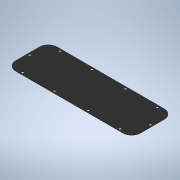
# Autodesk Inventor part: CAD_FPL_1050.000
Saved by Autodesk Inventor 2021 (Build 250183000, 183)
## iProperties
Created: 2025-07-29
Part Number: CAD_FPL_1050.000
Material: Generic
Catalog Web Link: www.cadenas.de
Description: Gland plate AX-Compact enclosures
Vendor: RITTAL
Document SubType Name: Modeling
Designer: psAdmin
Manufacturer: RITTAL
Mass: 97.9753 g
Surface Area: 1326.79 cm^2
Volume: 97.9753 cm^3
Density: 1 g/cm^3
Appearance: PSOLRGB-175-175-175
Category: PARTsolutions
Company: RITTAL
Title: CAD_FPL_1050.000
Author: Cadenas PARTsolutions
Comments: Compact enclosures
PSOL_IDENT_0: {$CADENAS_DATA/23d-libs/rittal/schaltschranksys/ausbauteile_cad/flanschplatten/ae_2_0_sep_fpl.prj},1
PSOL_IDENT_1: 81 {VTYP=3D},{NB=CAD_FPL_1050.000},{LINA=CAD_FPL_1050.000},{NN=Gland plate AX},{DATE=28.04.2025 21:1
PSOL_IDENT_2: 0:23},{GEOMDATE=11.04.2025 07:45:17},{VERSION=},{LINEID=180},{WBVAR=},{WBNUMERIC=}  {NB=CAD_FPL_1050
PSOL_IDENT_3: .000},{LINA=CAD_FPL_1050.000},{KT=DUMMY},{BEST=CAD_FPL_1050.000},{DETAIL=1},{VERS=4},{D=447},{E=149}
PSOL_IDENT_4: ,{BEZ1=Neues Kompaktgehäuse},{BEZ2=Stahlblech},{BEZ3=eintürig},{TUER=1},{B=500},{H=500},{T=210},{F=4
PSOL_IDENT_5: 50},{G=475},{B1=500},{B3=460.000},{B4=383.000},{B5=411.000},{BB5=0.000},{H1=500},{H3=460.000},{H4=85
PSOL_IDENT_6: .000},{H5=113.000},{HH5=4.000},{T5=93.500},{R1=31.000},{R2=8.000},{T1=210},{F1=450},{G1=475},{ST=MIN
PSOL_IDENT_7: },{VERS3=0},{CNSECLASS51=27-18-01-02},{CNSECLASS70=27-18-01-01},{CNSECLASS80=27-18-01-01},{CNSETIM40=
PSOL_IDENT_8: EC000261},{S=1.25},{W=500.000},{W1=456.500},{W2=400.000},{HH=500.000},{HH1=456.500},{HH2=450.000},{H
PSOL_IDENT_9: H3=375.000},{D1=204.300},{VERS1=1}
NB: CAD_FPL_1050.000
NN: Gland plate AX
NT: Compact enclosures
NBSYN: $BEST.
LINA: CAD_FPL_1050.000
CATALOG: Rittal
BEST: CAD_FPL_1050.000
D: 447
E: 149
SUPPLIER: RITTAL
ARTICLENO: CAD_FPL_1050.000
BOMINFO: CAD_FPL_1050.000
CREATOR: CADENAS GmbH
Autodesk Inventor part; units mm, degrees
(part 1 of 3)
sketch "Sketch_4" plane through (0, 0, 0) normal (0, 1, 0) x (1, 0, 0)
  arc A0 (-223.5, -42.5) -> (-191.5, -74.5) centre (-191.5, -42.5) ccw
  line L0 (-191.5, -74.5) -> (191.5, -74.5)
  arc A1 (191.5, -74.5) -> (223.5, -42.5) centre (191.5, -42.5) ccw
  line L1 (223.5, -42.5) -> (223.5, 42.5)
  arc A2 (223.5, 42.5) -> (191.5, 74.5) centre (191.5, 42.5) ccw
  line L2 (191.5, 74.5) -> (-191.5, 74.5)
  arc A3 (-191.5, 74.5) -> (-223.5, 42.5) centre (-191.5, 42.5) ccw
  line L3 (-223.5, 42.5) -> (-223.5, -42.5)
  circle A4 centre (215.5, 0) radius 3.6
  circle A5 centre (174, -66.5) radius 3.6
  circle A6 centre (174, 66.5) radius 3.6
  circle A7 centre (60, -66.5) radius 3.6
  circle A8 centre (60, 66.5) radius 3.6
  circle A9 centre (-60, -66.5) radius 3.6
  circle A10 centre (-60, 66.5) radius 3.6
  circle A11 centre (-174, -66.5) radius 3.6
  circle A12 centre (-174, 66.5) radius 3.6
  circle A13 centre (-215.5, 0) radius 3.6
  constraints: 14 centre point, 8 end point, 8 point on circle
extrude "Extrusion1" add sketch "Sketch_4" along normal blind 1.5
ref_plane "FP_XY" through (0, 0, 0) normal (0, -1, 0) x (1, 0, 0)
ref_plane "FP_YZ" through (0, 0, 0) normal (1, 0, 0) x (0, 0, 1)
ref_plane "FP_ZX" through (0, 0, 0) normal (0, 0, 1) x (0, -1, 0)
ref_plane "to_Bolt_1_XY" through (-250, 0, -250) normal (0, 1, 0) x (1, 0, 0)
ref_plane "to_Bolt_1_YZ" through (-250, 0, -250) normal (1, 0, 0) x (0, 0, -1)
ref_plane "to_Bolt_1_ZX" through (-250, 0, -250) normal (0, 0, -1) x (0, 1, 0)
ref_plane "to_Bolt_1_1_XY" through (-244, 0, -250) normal (0, 1, 0) x (1, 0, 0)
ref_plane "to_Bolt_1_1_YZ" through (-244, 0, -250) normal (1, 0, 0) x (0, 0, -1)
ref_plane "to_Bolt_1_1_ZX" through (-244, 0, -250) normal (0, 0, -1) x (0, 1, 0)
ref_plane "to_Bolt_1_10_XY" through (-228.4689, 0, -250) normal (0, 1, 0) x (1, 0, 0)
ref_plane "to_Bolt_1_10_YZ" through (-228.4689, 0, -250) normal (1, 0, 0) x (0, 0, -1)
ref_plane "to_Bolt_1_10_ZX" through (-228.4689, 0, -250) normal (0, 0, -1) x (0, 1, 0)
ref_plane "to_Bolt_1_100_XY" through (-13.1579, 0, -250) normal (0, 1, 0) x (1, 0, 0)
ref_plane "to_Bolt_1_100_YZ" through (-13.1579, 0, -250) normal (1, 0, 0) x (0, 0, -1)
ref_plane "to_Bolt_1_100_ZX" through (-13.1579, 0, -250) normal (0, 0, -1) x (0, 1, 0)
ref_plane "to_Bolt_1_101_XY" through (-10.7656, 0, -250) normal (0, 1, 0) x (1, 0, 0)
ref_plane "to_Bolt_1_101_YZ" through (-10.7656, 0, -250) normal (1, 0, 0) x (0, 0, -1)
ref_plane "to_Bolt_1_101_ZX" through (-10.7656, 0, -250) normal (0, 0, -1) x (0, 1, 0)
ref_plane "to_Bolt_1_102_XY" through (-8.3732, 0, -250) normal (0, 1, 0) x (1, 0, 0)
ref_plane "to_Bolt_1_102_YZ" through (-8.3732, 0, -250) normal (1, 0, 0) x (0, 0, -1)
ref_plane "to_Bolt_1_102_ZX" through (-8.3732, 0, -250) normal (0, 0, -1) x (0, 1, 0)
ref_plane "to_Bolt_1_103_XY" through (-5.9809, 0, -250) normal (0, 1, 0) x (1, 0, 0)
ref_plane "to_Bolt_1_103_YZ" through (-5.9809, 0, -250) normal (1, 0, 0) x (0, 0, -1)
ref_plane "to_Bolt_1_103_ZX" through (-5.9809, 0, -250) normal (0, 0, -1) x (0, 1, 0)
ref_plane "to_Bolt_1_104_XY" through (-3.5885, 0, -250) normal (0, 1, 0) x (1, 0, 0)
ref_plane "to_Bolt_1_104_YZ" through (-3.5885, 0, -250) normal (1, 0, 0) x (0, 0, -1)
ref_plane "to_Bolt_1_104_ZX" through (-3.5885, 0, -250) normal (0, 0, -1) x (0, 1, 0)
ref_plane "to_Bolt_1_105_XY" through (-1.1962, 0, -250) normal (0, 1, 0) x (1, 0, 0)
ref_plane "to_Bolt_1_105_YZ" through (-1.1962, 0, -250) normal (1, 0, 0) x (0, 0, -1)
ref_plane "to_Bolt_1_105_ZX" through (-1.1962, 0, -250) normal (0, 0, -1) x (0, 1, 0)
ref_plane "to_Bolt_1_106_XY" through (1.1962, 0, -250) normal (0, 1, 0) x (1, 0, 0)
ref_plane "to_Bolt_1_106_YZ" through (1.1962, 0, -250) normal (1, 0, 0) x (0, 0, -1)
ref_plane "to_Bolt_1_106_ZX" through (1.1962, 0, -250) normal (0, 0, -1) x (0, 1, 0)
ref_plane "to_Bolt_1_107_XY" through (3.5885, 0, -250) normal (0, 1, 0) x (1, 0, 0)
ref_plane "to_Bolt_1_107_YZ" through (3.5885, 0, -250) normal (1, 0, 0) x (0, 0, -1)
ref_plane "to_Bolt_1_107_ZX" through (3.5885, 0, -250) normal (0, 0, -1) x (0, 1, 0)
ref_plane "to_Bolt_1_108_XY" through (5.9809, 0, -250) normal (0, 1, 0) x (1, 0, 0)
ref_plane "to_Bolt_1_108_YZ" through (5.9809, 0, -250) normal (1, 0, 0) x (0, 0, -1)
ref_plane "to_Bolt_1_108_ZX" through (5.9809, 0, -250) normal (0, 0, -1) x (0, 1, 0)
ref_plane "to_Bolt_1_109_XY" through (8.3732, 0, -250) normal (0, 1, 0) x (1, 0, 0)
ref_plane "to_Bolt_1_109_YZ" through (8.3732, 0, -250) normal (1, 0, 0) x (0, 0, -1)
ref_plane "to_Bolt_1_109_ZX" through (8.3732, 0, -250) normal (0, 0, -1) x (0, 1, 0)
ref_plane "to_Bolt_1_11_XY" through (-226.0766, 0, -250) normal (0, 1, 0) x (1, 0, 0)
ref_plane "to_Bolt_1_11_YZ" through (-226.0766, 0, -250) normal (1, 0, 0) x (0, 0, -1)
ref_plane "to_Bolt_1_11_ZX" through (-226.0766, 0, -250) normal (0, 0, -1) x (0, 1, 0)
ref_plane "to_Bolt_1_110_XY" through (10.7656, 0, -250) normal (0, 1, 0) x (1, 0, 0)
ref_plane "to_Bolt_1_110_YZ" through (10.7656, 0, -250) normal (1, 0, 0) x (0, 0, -1)
ref_plane "to_Bolt_1_110_ZX" through (10.7656, 0, -250) normal (0, 0, -1) x (0, 1, 0)
ref_plane "to_Bolt_1_111_XY" through (13.1579, 0, -250) normal (0, 1, 0) x (1, 0, 0)
ref_plane "to_Bolt_1_111_YZ" through (13.1579, 0, -250) normal (1, 0, 0) x (0, 0, -1)
ref_plane "to_Bolt_1_111_ZX" through (13.1579, 0, -250) normal (0, 0, -1) x (0, 1, 0)
ref_plane "to_Bolt_1_112_XY" through (15.5502, 0, -250) normal (0, 1, 0) x (1, 0, 0)
ref_plane "to_Bolt_1_112_YZ" through (15.5502, 0, -250) normal (1, 0, 0) x (0, 0, -1)
ref_plane "to_Bolt_1_112_ZX" through (15.5502, 0, -250) normal (0, 0, -1) x (0, 1, 0)
ref_plane "to_Bolt_1_113_XY" through (17.9426, 0, -250) normal (0, 1, 0) x (1, 0, 0)
ref_plane "to_Bolt_1_113_YZ" through (17.9426, 0, -250) normal (1, 0, 0) x (0, 0, -1)
ref_plane "to_Bolt_1_113_ZX" through (17.9426, 0, -250) normal (0, 0, -1) x (0, 1, 0)
ref_plane "to_Bolt_1_114_XY" through (20.3349, 0, -250) normal (0, 1, 0) x (1, 0, 0)
ref_plane "to_Bolt_1_114_YZ" through (20.3349, 0, -250) normal (1, 0, 0) x (0, 0, -1)
ref_plane "to_Bolt_1_114_ZX" through (20.3349, 0, -250) normal (0, 0, -1) x (0, 1, 0)
ref_plane "to_Bolt_1_115_XY" through (22.7273, 0, -250) normal (0, 1, 0) x (1, 0, 0)
ref_plane "to_Bolt_1_115_YZ" through (22.7273, 0, -250) normal (1, 0, 0) x (0, 0, -1)
ref_plane "to_Bolt_1_115_ZX" through (22.7273, 0, -250) normal (0, 0, -1) x (0, 1, 0)
ref_plane "to_Bolt_1_116_XY" through (25.1196, 0, -250) normal (0, 1, 0) x (1, 0, 0)
ref_plane "to_Bolt_1_116_YZ" through (25.1196, 0, -250) normal (1, 0, 0) x (0, 0, -1)
ref_plane "to_Bolt_1_116_ZX" through (25.1196, 0, -250) normal (0, 0, -1) x (0, 1, 0)
ref_plane "to_Bolt_1_117_XY" through (27.512, 0, -250) normal (0, 1, 0) x (1, 0, 0)
ref_plane "to_Bolt_1_117_YZ" through (27.512, 0, -250) normal (1, 0, 0) x (0, 0, -1)
ref_plane "to_Bolt_1_117_ZX" through (27.512, 0, -250) normal (0, 0, -1) x (0, 1, 0)
ref_plane "to_Bolt_1_118_XY" through (29.9043, 0, -250) normal (0, 1, 0) x (1, 0, 0)
ref_plane "to_Bolt_1_118_YZ" through (29.9043, 0, -250) normal (1, 0, 0) x (0, 0, -1)
ref_plane "to_Bolt_1_118_ZX" through (29.9043, 0, -250) normal (0, 0, -1) x (0, 1, 0)
ref_plane "to_Bolt_1_119_XY" through (32.2967, 0, -250) normal (0, 1, 0) x (1, 0, 0)
ref_plane "to_Bolt_1_119_YZ" through (32.2967, 0, -250) normal (1, 0, 0) x (0, 0, -1)
ref_plane "to_Bolt_1_119_ZX" through (32.2967, 0, -250) normal (0, 0, -1) x (0, 1, 0)
ref_plane "to_Bolt_1_12_XY" through (-223.6842, 0, -250) normal (0, 1, 0) x (1, 0, 0)
ref_plane "to_Bolt_1_12_YZ" through (-223.6842, 0, -250) normal (1, 0, 0) x (0, 0, -1)
ref_plane "to_Bolt_1_12_ZX" through (-223.6842, 0, -250) normal (0, 0, -1) x (0, 1, 0)
ref_plane "to_Bolt_1_120_XY" through (34.689, 0, -250) normal (0, 1, 0) x (1, 0, 0)
ref_plane "to_Bolt_1_120_YZ" through (34.689, 0, -250) normal (1, 0, 0) x (0, 0, -1)
ref_plane "to_Bolt_1_120_ZX" through (34.689, 0, -250) normal (0, 0, -1) x (0, 1, 0)
ref_plane "to_Bolt_1_121_XY" through (37.0813, 0, -250) normal (0, 1, 0) x (1, 0, 0)
ref_plane "to_Bolt_1_121_YZ" through (37.0813, 0, -250) normal (1, 0, 0) x (0, 0, -1)
ref_plane "to_Bolt_1_121_ZX" through (37.0813, 0, -250) normal (0, 0, -1) x (0, 1, 0)
ref_plane "to_Bolt_1_122_XY" through (39.4737, 0, -250) normal (0, 1, 0) x (1, 0, 0)
ref_plane "to_Bolt_1_122_YZ" through (39.4737, 0, -250) normal (1, 0, 0) x (0, 0, -1)
ref_plane "to_Bolt_1_122_ZX" through (39.4737, 0, -250) normal (0, 0, -1) x (0, 1, 0)
ref_plane "to_Bolt_1_123_XY" through (41.866, 0, -250) normal (0, 1, 0) x (1, 0, 0)
ref_plane "to_Bolt_1_123_YZ" through (41.866, 0, -250) normal (1, 0, 0) x (0, 0, -1)
ref_plane "to_Bolt_1_123_ZX" through (41.866, 0, -250) normal (0, 0, -1) x (0, 1, 0)
ref_plane "to_Bolt_1_124_XY" through (44.2584, 0, -250) normal (0, 1, 0) x (1, 0, 0)
ref_plane "to_Bolt_1_124_YZ" through (44.2584, 0, -250) normal (1, 0, 0) x (0, 0, -1)
ref_plane "to_Bolt_1_124_ZX" through (44.2584, 0, -250) normal (0, 0, -1) x (0, 1, 0)
ref_plane "to_Bolt_1_125_XY" through (46.6507, 0, -250) normal (0, 1, 0) x (1, 0, 0)
ref_plane "to_Bolt_1_125_YZ" through (46.6507, 0, -250) normal (1, 0, 0) x (0, 0, -1)
ref_plane "to_Bolt_1_125_ZX" through (46.6507, 0, -250) normal (0, 0, -1) x (0, 1, 0)
ref_plane "to_Bolt_1_126_XY" through (49.0431, 0, -250) normal (0, 1, 0) x (1, 0, 0)
ref_plane "to_Bolt_1_126_YZ" through (49.0431, 0, -250) normal (1, 0, 0) x (0, 0, -1)
ref_plane "to_Bolt_1_126_ZX" through (49.0431, 0, -250) normal (0, 0, -1) x (0, 1, 0)
ref_plane "to_Bolt_1_127_XY" through (51.4354, 0, -250) normal (0, 1, 0) x (1, 0, 0)
ref_plane "to_Bolt_1_127_YZ" through (51.4354, 0, -250) normal (1, 0, 0) x (0, 0, -1)
ref_plane "to_Bolt_1_127_ZX" through (51.4354, 0, -250) normal (0, 0, -1) x (0, 1, 0)
ref_plane "to_Bolt_1_128_XY" through (53.8278, 0, -250) normal (0, 1, 0) x (1, 0, 0)
ref_plane "to_Bolt_1_128_YZ" through (53.8278, 0, -250) normal (1, 0, 0) x (0, 0, -1)
ref_plane "to_Bolt_1_128_ZX" through (53.8278, 0, -250) normal (0, 0, -1) x (0, 1, 0)
ref_plane "to_Bolt_1_129_XY" through (56.2201, 0, -250) normal (0, 1, 0) x (1, 0, 0)
ref_plane "to_Bolt_1_129_YZ" through (56.2201, 0, -250) normal (1, 0, 0) x (0, 0, -1)
ref_plane "to_Bolt_1_129_ZX" through (56.2201, 0, -250) normal (0, 0, -1) x (0, 1, 0)
ref_plane "to_Bolt_1_13_XY" through (-221.2919, 0, -250) normal (0, 1, 0) x (1, 0, 0)
ref_plane "to_Bolt_1_13_YZ" through (-221.2919, 0, -250) normal (1, 0, 0) x (0, 0, -1)
ref_plane "to_Bolt_1_13_ZX" through (-221.2919, 0, -250) normal (0, 0, -1) x (0, 1, 0)
ref_plane "to_Bolt_1_130_XY" through (58.6124, 0, -250) normal (0, 1, 0) x (1, 0, 0)
ref_plane "to_Bolt_1_130_YZ" through (58.6124, 0, -250) normal (1, 0, 0) x (0, 0, -1)
ref_plane "to_Bolt_1_130_ZX" through (58.6124, 0, -250) normal (0, 0, -1) x (0, 1, 0)
ref_plane "to_Bolt_1_131_XY" through (61.0048, 0, -250) normal (0, 1, 0) x (1, 0, 0)
ref_plane "to_Bolt_1_131_YZ" through (61.0048, 0, -250) normal (1, 0, 0) x (0, 0, -1)
ref_plane "to_Bolt_1_131_ZX" through (61.0048, 0, -250) normal (0, 0, -1) x (0, 1, 0)
ref_plane "to_Bolt_1_132_XY" through (63.3971, 0, -250) normal (0, 1, 0) x (1, 0, 0)
ref_plane "to_Bolt_1_132_YZ" through (63.3971, 0, -250) normal (1, 0, 0) x (0, 0, -1)
ref_plane "to_Bolt_1_132_ZX" through (63.3971, 0, -250) normal (0, 0, -1) x (0, 1, 0)
ref_plane "to_Bolt_1_133_XY" through (65.7895, 0, -250) normal (0, 1, 0) x (1, 0, 0)
ref_plane "to_Bolt_1_133_YZ" through (65.7895, 0, -250) normal (1, 0, 0) x (0, 0, -1)
ref_plane "to_Bolt_1_133_ZX" through (65.7895, 0, -250) normal (0, 0, -1) x (0, 1, 0)
ref_plane "to_Bolt_1_134_XY" through (68.1818, 0, -250) normal (0, 1, 0) x (1, 0, 0)
ref_plane "to_Bolt_1_134_YZ" through (68.1818, 0, -250) normal (1, 0, 0) x (0, 0, -1)
ref_plane "to_Bolt_1_134_ZX" through (68.1818, 0, -250) normal (0, 0, -1) x (0, 1, 0)
ref_plane "to_Bolt_1_135_XY" through (70.5742, 0, -250) normal (0, 1, 0) x (1, 0, 0)
ref_plane "to_Bolt_1_135_YZ" through (70.5742, 0, -250) normal (1, 0, 0) x (0, 0, -1)
ref_plane "to_Bolt_1_135_ZX" through (70.5742, 0, -250) normal (0, 0, -1) x (0, 1, 0)
ref_plane "to_Bolt_1_136_XY" through (72.9665, 0, -250) normal (0, 1, 0) x (1, 0, 0)
ref_plane "to_Bolt_1_136_YZ" through (72.9665, 0, -250) normal (1, 0, 0) x (0, 0, -1)
ref_plane "to_Bolt_1_136_ZX" through (72.9665, 0, -250) normal (0, 0, -1) x (0, 1, 0)
ref_plane "to_Bolt_1_137_XY" through (75.3589, 0, -250) normal (0, 1, 0) x (1, 0, 0)
ref_plane "to_Bolt_1_137_YZ" through (75.3589, 0, -250) normal (1, 0, 0) x (0, 0, -1)
ref_plane "to_Bolt_1_137_ZX" through (75.3589, 0, -250) normal (0, 0, -1) x (0, 1, 0)
ref_plane "to_Bolt_1_138_XY" through (77.7512, 0, -250) normal (0, 1, 0) x (1, 0, 0)
ref_plane "to_Bolt_1_138_YZ" through (77.7512, 0, -250) normal (1, 0, 0) x (0, 0, -1)
ref_plane "to_Bolt_1_138_ZX" through (77.7512, 0, -250) normal (0, 0, -1) x (0, 1, 0)
ref_plane "to_Bolt_1_139_XY" through (80.1435, 0, -250) normal (0, 1, 0) x (1, 0, 0)
ref_plane "to_Bolt_1_139_YZ" through (80.1435, 0, -250) normal (1, 0, 0) x (0, 0, -1)
ref_plane "to_Bolt_1_139_ZX" through (80.1435, 0, -250) normal (0, 0, -1) x (0, 1, 0)
ref_plane "to_Bolt_1_14_XY" through (-218.8995, 0, -250) normal (0, 1, 0) x (1, 0, 0)
ref_plane "to_Bolt_1_14_YZ" through (-218.8995, 0, -250) normal (1, 0, 0) x (0, 0, -1)
ref_plane "to_Bolt_1_14_ZX" through (-218.8995, 0, -250) normal (0, 0, -1) x (0, 1, 0)
ref_plane "to_Bolt_1_140_XY" through (82.5359, 0, -250) normal (0, 1, 0) x (1, 0, 0)
ref_plane "to_Bolt_1_140_YZ" through (82.5359, 0, -250) normal (1, 0, 0) x (0, 0, -1)
ref_plane "to_Bolt_1_140_ZX" through (82.5359, 0, -250) normal (0, 0, -1) x (0, 1, 0)
ref_plane "to_Bolt_1_141_XY" through (84.9282, 0, -250) normal (0, 1, 0) x (1, 0, 0)
ref_plane "to_Bolt_1_141_YZ" through (84.9282, 0, -250) normal (1, 0, 0) x (0, 0, -1)
ref_plane "to_Bolt_1_141_ZX" through (84.9282, 0, -250) normal (0, 0, -1) x (0, 1, 0)
ref_plane "to_Bolt_1_142_XY" through (87.3206, 0, -250) normal (0, 1, 0) x (1, 0, 0)
ref_plane "to_Bolt_1_142_YZ" through (87.3206, 0, -250) normal (1, 0, 0) x (0, 0, -1)
ref_plane "to_Bolt_1_142_ZX" through (87.3206, 0, -250) normal (0, 0, -1) x (0, 1, 0)
ref_plane "to_Bolt_1_143_XY" through (89.7129, 0, -250) normal (0, 1, 0) x (1, 0, 0)
ref_plane "to_Bolt_1_143_YZ" through (89.7129, 0, -250) normal (1, 0, 0) x (0, 0, -1)
ref_plane "to_Bolt_1_143_ZX" through (89.7129, 0, -250) normal (0, 0, -1) x (0, 1, 0)
ref_plane "to_Bolt_1_144_XY" through (92.1053, 0, -250) normal (0, 1, 0) x (1, 0, 0)
ref_plane "to_Bolt_1_144_YZ" through (92.1053, 0, -250) normal (1, 0, 0) x (0, 0, -1)
ref_plane "to_Bolt_1_144_ZX" through (92.1053, 0, -250) normal (0, 0, -1) x (0, 1, 0)
ref_plane "to_Bolt_1_145_XY" through (94.4976, 0, -250) normal (0, 1, 0) x (1, 0, 0)
ref_plane "to_Bolt_1_145_YZ" through (94.4976, 0, -250) normal (1, 0, 0) x (0, 0, -1)
ref_plane "to_Bolt_1_145_ZX" through (94.4976, 0, -250) normal (0, 0, -1) x (0, 1, 0)
ref_plane "to_Bolt_1_146_XY" through (96.89, 0, -250) normal (0, 1, 0) x (1, 0, 0)
ref_plane "to_Bolt_1_146_YZ" through (96.89, 0, -250) normal (1, 0, 0) x (0, 0, -1)
ref_plane "to_Bolt_1_146_ZX" through (96.89, 0, -250) normal (0, 0, -1) x (0, 1, 0)
ref_plane "to_Bolt_1_147_XY" through (99.2823, 0, -250) normal (0, 1, 0) x (1, 0, 0)
ref_plane "to_Bolt_1_147_YZ" through (99.2823, 0, -250) normal (1, 0, 0) x (0, 0, -1)
ref_plane "to_Bolt_1_147_ZX" through (99.2823, 0, -250) normal (0, 0, -1) x (0, 1, 0)
ref_plane "to_Bolt_1_148_XY" through (101.6746, 0, -250) normal (0, 1, 0) x (1, 0, 0)
ref_plane "to_Bolt_1_148_YZ" through (101.6746, 0, -250) normal (1, 0, 0) x (0, 0, -1)
ref_plane "to_Bolt_1_148_ZX" through (101.6746, 0, -250) normal (0, 0, -1) x (0, 1, 0)
ref_plane "to_Bolt_1_149_XY" through (104.067, 0, -250) normal (0, 1, 0) x (1, 0, 0)
ref_plane "to_Bolt_1_149_YZ" through (104.067, 0, -250) normal (1, 0, 0) x (0, 0, -1)
ref_plane "to_Bolt_1_149_ZX" through (104.067, 0, -250) normal (0, 0, -1) x (0, 1, 0)
ref_plane "to_Bolt_1_15_XY" through (-216.5072, 0, -250) normal (0, 1, 0) x (1, 0, 0)
ref_plane "to_Bolt_1_15_YZ" through (-216.5072, 0, -250) normal (1, 0, 0) x (0, 0, -1)
ref_plane "to_Bolt_1_15_ZX" through (-216.5072, 0, -250) normal (0, 0, -1) x (0, 1, 0)
ref_plane "to_Bolt_1_150_XY" through (106.4593, 0, -250) normal (0, 1, 0) x (1, 0, 0)
ref_plane "to_Bolt_1_150_YZ" through (106.4593, 0, -250) normal (1, 0, 0) x (0, 0, -1)
ref_plane "to_Bolt_1_150_ZX" through (106.4593, 0, -250) normal (0, 0, -1) x (0, 1, 0)
ref_plane "to_Bolt_1_151_XY" through (108.8517, 0, -250) normal (0, 1, 0) x (1, 0, 0)
ref_plane "to_Bolt_1_151_YZ" through (108.8517, 0, -250) normal (1, 0, 0) x (0, 0, -1)
ref_plane "to_Bolt_1_151_ZX" through (108.8517, 0, -250) normal (0, 0, -1) x (0, 1, 0)
ref_plane "to_Bolt_1_152_XY" through (111.244, 0, -250) normal (0, 1, 0) x (1, 0, 0)
ref_plane "to_Bolt_1_152_YZ" through (111.244, 0, -250) normal (1, 0, 0) x (0, 0, -1)
ref_plane "to_Bolt_1_152_ZX" through (111.244, 0, -250) normal (0, 0, -1) x (0, 1, 0)
ref_plane "to_Bolt_1_153_XY" through (113.6364, 0, -250) normal (0, 1, 0) x (1, 0, 0)
ref_plane "to_Bolt_1_153_YZ" through (113.6364, 0, -250) normal (1, 0, 0) x (0, 0, -1)
ref_plane "to_Bolt_1_153_ZX" through (113.6364, 0, -250) normal (0, 0, -1) x (0, 1, 0)
ref_plane "to_Bolt_1_154_XY" through (116.0287, 0, -250) normal (0, 1, 0) x (1, 0, 0)
ref_plane "to_Bolt_1_154_YZ" through (116.0287, 0, -250) normal (1, 0, 0) x (0, 0, -1)
ref_plane "to_Bolt_1_154_ZX" through (116.0287, 0, -250) normal (0, 0, -1) x (0, 1, 0)
ref_plane "to_Bolt_1_155_XY" through (118.4211, 0, -250) normal (0, 1, 0) x (1, 0, 0)
ref_plane "to_Bolt_1_155_YZ" through (118.4211, 0, -250) normal (1, 0, 0) x (0, 0, -1)
ref_plane "to_Bolt_1_155_ZX" through (118.4211, 0, -250) normal (0, 0, -1) x (0, 1, 0)
ref_plane "to_Bolt_1_156_XY" through (120.8134, 0, -250) normal (0, 1, 0) x (1, 0, 0)
ref_plane "to_Bolt_1_156_YZ" through (120.8134, 0, -250) normal (1, 0, 0) x (0, 0, -1)
ref_plane "to_Bolt_1_156_ZX" through (120.8134, 0, -250) normal (0, 0, -1) x (0, 1, 0)
ref_plane "to_Bolt_1_157_XY" through (123.2057, 0, -250) normal (0, 1, 0) x (1, 0, 0)
ref_plane "to_Bolt_1_157_YZ" through (123.2057, 0, -250) normal (1, 0, 0) x (0, 0, -1)
ref_plane "to_Bolt_1_157_ZX" through (123.2057, 0, -250) normal (0, 0, -1) x (0, 1, 0)
ref_plane "to_Bolt_1_158_XY" through (125.5981, 0, -250) normal (0, 1, 0) x (1, 0, 0)
ref_plane "to_Bolt_1_158_YZ" through (125.5981, 0, -250) normal (1, 0, 0) x (0, 0, -1)
ref_plane "to_Bolt_1_158_ZX" through (125.5981, 0, -250) normal (0, 0, -1) x (0, 1, 0)
ref_plane "to_Bolt_1_159_XY" through (127.9904, 0, -250) normal (0, 1, 0) x (1, 0, 0)
ref_plane "to_Bolt_1_159_YZ" through (127.9904, 0, -250) normal (1, 0, 0) x (0, 0, -1)
ref_plane "to_Bolt_1_159_ZX" through (127.9904, 0, -250) normal (0, 0, -1) x (0, 1, 0)
ref_plane "to_Bolt_1_16_XY" through (-214.1148, 0, -250) normal (0, 1, 0) x (1, 0, 0)
ref_plane "to_Bolt_1_16_YZ" through (-214.1148, 0, -250) normal (1, 0, 0) x (0, 0, -1)
ref_plane "to_Bolt_1_16_ZX" through (-214.1148, 0, -250) normal (0, 0, -1) x (0, 1, 0)
ref_plane "to_Bolt_1_160_XY" through (130.3828, 0, -250) normal (0, 1, 0) x (1, 0, 0)
ref_plane "to_Bolt_1_160_YZ" through (130.3828, 0, -250) normal (1, 0, 0) x (0, 0, -1)
ref_plane "to_Bolt_1_160_ZX" through (130.3828, 0, -250) normal (0, 0, -1) x (0, 1, 0)
ref_plane "to_Bolt_1_161_XY" through (132.7751, 0, -250) normal (0, 1, 0) x (1, 0, 0)
ref_plane "to_Bolt_1_161_YZ" through (132.7751, 0, -250) normal (1, 0, 0) x (0, 0, -1)
ref_plane "to_Bolt_1_161_ZX" through (132.7751, 0, -250) normal (0, 0, -1) x (0, 1, 0)
ref_plane "to_Bolt_1_162_XY" through (135.1675, 0, -250) normal (0, 1, 0) x (1, 0, 0)
ref_plane "to_Bolt_1_162_YZ" through (135.1675, 0, -250) normal (1, 0, 0) x (0, 0, -1)
ref_plane "to_Bolt_1_162_ZX" through (135.1675, 0, -250) normal (0, 0, -1) x (0, 1, 0)
ref_plane "to_Bolt_1_163_XY" through (137.5598, 0, -250) normal (0, 1, 0) x (1, 0, 0)
ref_plane "to_Bolt_1_163_YZ" through (137.5598, 0, -250) normal (1, 0, 0) x (0, 0, -1)
ref_plane "to_Bolt_1_163_ZX" through (137.5598, 0, -250) normal (0, 0, -1) x (0, 1, 0)
ref_plane "to_Bolt_1_164_XY" through (139.9522, 0, -250) normal (0, 1, 0) x (1, 0, 0)
ref_plane "to_Bolt_1_164_YZ" through (139.9522, 0, -250) normal (1, 0, 0) x (0, 0, -1)
ref_plane "to_Bolt_1_164_ZX" through (139.9522, 0, -250) normal (0, 0, -1) x (0, 1, 0)
ref_plane "to_Bolt_1_165_XY" through (142.3445, 0, -250) normal (0, 1, 0) x (1, 0, 0)
ref_plane "to_Bolt_1_165_YZ" through (142.3445, 0, -250) normal (1, 0, 0) x (0, 0, -1)
ref_plane "to_Bolt_1_165_ZX" through (142.3445, 0, -250) normal (0, 0, -1) x (0, 1, 0)
ref_plane "to_Bolt_1_166_XY" through (144.7368, 0, -250) normal (0, 1, 0) x (1, 0, 0)
ref_plane "to_Bolt_1_166_YZ" through (144.7368, 0, -250) normal (1, 0, 0) x (0, 0, -1)
ref_plane "to_Bolt_1_166_ZX" through (144.7368, 0, -250) normal (0, 0, -1) x (0, 1, 0)
ref_plane "to_Bolt_1_167_XY" through (147.1292, 0, -250) normal (0, 1, 0) x (1, 0, 0)
ref_plane "to_Bolt_1_167_YZ" through (147.1292, 0, -250) normal (1, 0, 0) x (0, 0, -1)
ref_plane "to_Bolt_1_167_ZX" through (147.1292, 0, -250) normal (0, 0, -1) x (0, 1, 0)
ref_plane "to_Bolt_1_168_XY" through (149.5215, 0, -250) normal (0, 1, 0) x (1, 0, 0)
ref_plane "to_Bolt_1_168_YZ" through (149.5215, 0, -250) normal (1, 0, 0) x (0, 0, -1)
ref_plane "to_Bolt_1_168_ZX" through (149.5215, 0, -250) normal (0, 0, -1) x (0, 1, 0)
ref_plane "to_Bolt_1_169_XY" through (151.9139, 0, -250) normal (0, 1, 0) x (1, 0, 0)
ref_plane "to_Bolt_1_169_YZ" through (151.9139, 0, -250) normal (1, 0, 0) x (0, 0, -1)
ref_plane "to_Bolt_1_169_ZX" through (151.9139, 0, -250) normal (0, 0, -1) x (0, 1, 0)
ref_plane "to_Bolt_1_17_XY" through (-211.7225, 0, -250) normal (0, 1, 0) x (1, 0, 0)
ref_plane "to_Bolt_1_17_YZ" through (-211.7225, 0, -250) normal (1, 0, 0) x (0, 0, -1)
ref_plane "to_Bolt_1_17_ZX" through (-211.7225, 0, -250) normal (0, 0, -1) x (0, 1, 0)
ref_plane "to_Bolt_1_170_XY" through (154.3062, 0, -250) normal (0, 1, 0) x (1, 0, 0)
ref_plane "to_Bolt_1_170_YZ" through (154.3062, 0, -250) normal (1, 0, 0) x (0, 0, -1)
ref_plane "to_Bolt_1_170_ZX" through (154.3062, 0, -250) normal (0, 0, -1) x (0, 1, 0)
ref_plane "to_Bolt_1_171_XY" through (156.6986, 0, -250) normal (0, 1, 0) x (1, 0, 0)
ref_plane "to_Bolt_1_171_YZ" through (156.6986, 0, -250) normal (1, 0, 0) x (0, 0, -1)
ref_plane "to_Bolt_1_171_ZX" through (156.6986, 0, -250) normal (0, 0, -1) x (0, 1, 0)
ref_plane "to_Bolt_1_172_XY" through (159.0909, 0, -250) normal (0, 1, 0) x (1, 0, 0)
ref_plane "to_Bolt_1_172_YZ" through (159.0909, 0, -250) normal (1, 0, 0) x (0, 0, -1)
ref_plane "to_Bolt_1_172_ZX" through (159.0909, 0, -250) normal (0, 0, -1) x (0, 1, 0)
ref_plane "to_Bolt_1_173_XY" through (161.4833, 0, -250) normal (0, 1, 0) x (1, 0, 0)
ref_plane "to_Bolt_1_173_YZ" through (161.4833, 0, -250) normal (1, 0, 0) x (0, 0, -1)
ref_plane "to_Bolt_1_173_ZX" through (161.4833, 0, -250) normal (0, 0, -1) x (0, 1, 0)
ref_plane "to_Bolt_1_174_XY" through (163.8756, 0, -250) normal (0, 1, 0) x (1, 0, 0)
ref_plane "to_Bolt_1_174_YZ" through (163.8756, 0, -250) normal (1, 0, 0) x (0, 0, -1)
ref_plane "to_Bolt_1_174_ZX" through (163.8756, 0, -250) normal (0, 0, -1) x (0, 1, 0)
ref_plane "to_Bolt_1_175_XY" through (166.2679, 0, -250) normal (0, 1, 0) x (1, 0, 0)
ref_plane "to_Bolt_1_175_YZ" through (166.2679, 0, -250) normal (1, 0, 0) x (0, 0, -1)
ref_plane "to_Bolt_1_175_ZX" through (166.2679, 0, -250) normal (0, 0, -1) x (0, 1, 0)
ref_plane "to_Bolt_1_176_XY" through (168.6603, 0, -250) normal (0, 1, 0) x (1, 0, 0)
ref_plane "to_Bolt_1_176_YZ" through (168.6603, 0, -250) normal (1, 0, 0) x (0, 0, -1)
ref_plane "to_Bolt_1_176_ZX" through (168.6603, 0, -250) normal (0, 0, -1) x (0, 1, 0)
ref_plane "to_Bolt_1_177_XY" through (171.0526, 0, -250) normal (0, 1, 0) x (1, 0, 0)
ref_plane "to_Bolt_1_177_YZ" through (171.0526, 0, -250) normal (1, 0, 0) x (0, 0, -1)
ref_plane "to_Bolt_1_177_ZX" through (171.0526, 0, -250) normal (0, 0, -1) x (0, 1, 0)
ref_plane "to_Bolt_1_178_XY" through (173.445, 0, -250) normal (0, 1, 0) x (1, 0, 0)
ref_plane "to_Bolt_1_178_YZ" through (173.445, 0, -250) normal (1, 0, 0) x (0, 0, -1)
ref_plane "to_Bolt_1_178_ZX" through (173.445, 0, -250) normal (0, 0, -1) x (0, 1, 0)
ref_plane "to_Bolt_1_179_XY" through (175.8373, 0, -250) normal (0, 1, 0) x (1, 0, 0)
ref_plane "to_Bolt_1_179_YZ" through (175.8373, 0, -250) normal (1, 0, 0) x (0, 0, -1)
ref_plane "to_Bolt_1_179_ZX" through (175.8373, 0, -250) normal (0, 0, -1) x (0, 1, 0)
ref_plane "to_Bolt_1_18_XY" through (-209.3301, 0, -250) normal (0, 1, 0) x (1, 0, 0)
ref_plane "to_Bolt_1_18_YZ" through (-209.3301, 0, -250) normal (1, 0, 0) x (0, 0, -1)
ref_plane "to_Bolt_1_18_ZX" through (-209.3301, 0, -250) normal (0, 0, -1) x (0, 1, 0)
ref_plane "to_Bolt_1_180_XY" through (178.2297, 0, -250) normal (0, 1, 0) x (1, 0, 0)
ref_plane "to_Bolt_1_180_YZ" through (178.2297, 0, -250) normal (1, 0, 0) x (0, 0, -1)
ref_plane "to_Bolt_1_180_ZX" through (178.2297, 0, -250) normal (0, 0, -1) x (0, 1, 0)
ref_plane "to_Bolt_1_181_XY" through (180.622, 0, -250) normal (0, 1, 0) x (1, 0, 0)
ref_plane "to_Bolt_1_181_YZ" through (180.622, 0, -250) normal (1, 0, 0) x (0, 0, -1)
ref_plane "to_Bolt_1_181_ZX" through (180.622, 0, -250) normal (0, 0, -1) x (0, 1, 0)
ref_plane "to_Bolt_1_182_XY" through (183.0144, 0, -250) normal (0, 1, 0) x (1, 0, 0)
ref_plane "to_Bolt_1_182_YZ" through (183.0144, 0, -250) normal (1, 0, 0) x (0, 0, -1)
ref_plane "to_Bolt_1_182_ZX" through (183.0144, 0, -250) normal (0, 0, -1) x (0, 1, 0)
ref_plane "to_Bolt_1_183_XY" through (185.4067, 0, -250) normal (0, 1, 0) x (1, 0, 0)
ref_plane "to_Bolt_1_183_YZ" through (185.4067, 0, -250) normal (1, 0, 0) x (0, 0, -1)
ref_plane "to_Bolt_1_183_ZX" through (185.4067, 0, -250) normal (0, 0, -1) x (0, 1, 0)
ref_plane "to_Bolt_1_184_XY" through (187.799, 0, -250) normal (0, 1, 0) x (1, 0, 0)
ref_plane "to_Bolt_1_184_YZ" through (187.799, 0, -250) normal (1, 0, 0) x (0, 0, -1)
ref_plane "to_Bolt_1_184_ZX" through (187.799, 0, -250) normal (0, 0, -1) x (0, 1, 0)
ref_plane "to_Bolt_1_185_XY" through (190.1914, 0, -250) normal (0, 1, 0) x (1, 0, 0)
ref_plane "to_Bolt_1_185_YZ" through (190.1914, 0, -250) normal (1, 0, 0) x (0, 0, -1)
ref_plane "to_Bolt_1_185_ZX" through (190.1914, 0, -250) normal (0, 0, -1) x (0, 1, 0)
ref_plane "to_Bolt_1_186_XY" through (192.5837, 0, -250) normal (0, 1, 0) x (1, 0, 0)
ref_plane "to_Bolt_1_186_YZ" through (192.5837, 0, -250) normal (1, 0, 0) x (0, 0, -1)
ref_plane "to_Bolt_1_186_ZX" through (192.5837, 0, -250) normal (0, 0, -1) x (0, 1, 0)
ref_plane "to_Bolt_1_187_XY" through (194.9761, 0, -250) normal (0, 1, 0) x (1, 0, 0)
ref_plane "to_Bolt_1_187_YZ" through (194.9761, 0, -250) normal (1, 0, 0) x (0, 0, -1)
ref_plane "to_Bolt_1_187_ZX" through (194.9761, 0, -250) normal (0, 0, -1) x (0, 1, 0)
ref_plane "to_Bolt_1_188_XY" through (197.3684, 0, -250) normal (0, 1, 0) x (1, 0, 0)
ref_plane "to_Bolt_1_188_YZ" through (197.3684, 0, -250) normal (1, 0, 0) x (0, 0, -1)
ref_plane "to_Bolt_1_188_ZX" through (197.3684, 0, -250) normal (0, 0, -1) x (0, 1, 0)
ref_plane "to_Bolt_1_189_XY" through (199.7608, 0, -250) normal (0, 1, 0) x (1, 0, 0)
ref_plane "to_Bolt_1_189_YZ" through (199.7608, 0, -250) normal (1, 0, 0) x (0, 0, -1)
ref_plane "to_Bolt_1_189_ZX" through (199.7608, 0, -250) normal (0, 0, -1) x (0, 1, 0)
ref_plane "to_Bolt_1_19_XY" through (-206.9378, 0, -250) normal (0, 1, 0) x (1, 0, 0)
ref_plane "to_Bolt_1_19_YZ" through (-206.9378, 0, -250) normal (1, 0, 0) x (0, 0, -1)
ref_plane "to_Bolt_1_19_ZX" through (-206.9378, 0, -250) normal (0, 0, -1) x (0, 1, 0)
ref_plane "to_Bolt_1_190_XY" through (202.1531, 0, -250) normal (0, 1, 0) x (1, 0, 0)
ref_plane "to_Bolt_1_190_YZ" through (202.1531, 0, -250) normal (1, 0, 0) x (0, 0, -1)
ref_plane "to_Bolt_1_190_ZX" through (202.1531, 0, -250) normal (0, 0, -1) x (0, 1, 0)
ref_plane "to_Bolt_1_191_XY" through (204.5455, 0, -250) normal (0, 1, 0) x (1, 0, 0)
ref_plane "to_Bolt_1_191_YZ" through (204.5455, 0, -250) normal (1, 0, 0) x (0, 0, -1)
ref_plane "to_Bolt_1_191_ZX" through (204.5455, 0, -250) normal (0, 0, -1) x (0, 1, 0)
ref_plane "to_Bolt_1_192_XY" through (206.9378, 0, -250) normal (0, 1, 0) x (1, 0, 0)
ref_plane "to_Bolt_1_192_YZ" through (206.9378, 0, -250) normal (1, 0, 0) x (0, 0, -1)
ref_plane "to_Bolt_1_192_ZX" through (206.9378, 0, -250) normal (0, 0, -1) x (0, 1, 0)
ref_plane "to_Bolt_1_193_XY" through (209.3301, 0, -250) normal (0, 1, 0) x (1, 0, 0)
ref_plane "to_Bolt_1_193_YZ" through (209.3301, 0, -250) normal (1, 0, 0) x (0, 0, -1)
ref_plane "to_Bolt_1_193_ZX" through (209.3301, 0, -250) normal (0, 0, -1) x (0, 1, 0)
ref_plane "to_Bolt_1_194_XY" through (211.7225, 0, -250) normal (0, 1, 0) x (1, 0, 0)
ref_plane "to_Bolt_1_194_YZ" through (211.7225, 0, -250) normal (1, 0, 0) x (0, 0, -1)
ref_plane "to_Bolt_1_194_ZX" through (211.7225, 0, -250) normal (0, 0, -1) x (0, 1, 0)
ref_plane "to_Bolt_1_195_XY" through (214.1148, 0, -250) normal (0, 1, 0) x (1, 0, 0)
ref_plane "to_Bolt_1_195_YZ" through (214.1148, 0, -250) normal (1, 0, 0) x (0, 0, -1)
ref_plane "to_Bolt_1_195_ZX" through (214.1148, 0, -250) normal (0, 0, -1) x (0, 1, 0)
ref_plane "to_Bolt_1_196_XY" through (216.5072, 0, -250) normal (0, 1, 0) x (1, 0, 0)
ref_plane "to_Bolt_1_196_YZ" through (216.5072, 0, -250) normal (1, 0, 0) x (0, 0, -1)
ref_plane "to_Bolt_1_196_ZX" through (216.5072, 0, -250) normal (0, 0, -1) x (0, 1, 0)
ref_plane "to_Bolt_1_197_XY" through (218.8995, 0, -250) normal (0, 1, 0) x (1, 0, 0)
ref_plane "to_Bolt_1_197_YZ" through (218.8995, 0, -250) normal (1, 0, 0) x (0, 0, -1)
ref_plane "to_Bolt_1_197_ZX" through (218.8995, 0, -250) normal (0, 0, -1) x (0, 1, 0)
ref_plane "to_Bolt_1_198_XY" through (221.2919, 0, -250) normal (0, 1, 0) x (1, 0, 0)
ref_plane "to_Bolt_1_198_YZ" through (221.2919, 0, -250) normal (1, 0, 0) x (0, 0, -1)
ref_plane "to_Bolt_1_198_ZX" through (221.2919, 0, -250) normal (0, 0, -1) x (0, 1, 0)
ref_plane "to_Bolt_1_199_XY" through (223.6842, 0, -250) normal (0, 1, 0) x (1, 0, 0)
ref_plane "to_Bolt_1_199_YZ" through (223.6842, 0, -250) normal (1, 0, 0) x (0, 0, -1)
ref_plane "to_Bolt_1_199_ZX" through (223.6842, 0, -250) normal (0, 0, -1) x (0, 1, 0)
ref_plane "to_Bolt_1_2_XY" through (-247.6077, 0, -250) normal (0, 1, 0) x (1, 0, 0)
ref_plane "to_Bolt_1_2_YZ" through (-247.6077, 0, -250) normal (1, 0, 0) x (0, 0, -1)
ref_plane "to_Bolt_1_2_ZX" through (-247.6077, 0, -250) normal (0, 0, -1) x (0, 1, 0)
ref_plane "to_Bolt_1_20_XY" through (-204.5455, 0, -250) normal (0, 1, 0) x (1, 0, 0)
ref_plane "to_Bolt_1_20_YZ" through (-204.5455, 0, -250) normal (1, 0, 0) x (0, 0, -1)
ref_plane "to_Bolt_1_20_ZX" through (-204.5455, 0, -250) normal (0, 0, -1) x (0, 1, 0)
ref_plane "to_Bolt_1_200_XY" through (226.0766, 0, -250) normal (0, 1, 0) x (1, 0, 0)
ref_plane "to_Bolt_1_200_YZ" through (226.0766, 0, -250) normal (1, 0, 0) x (0, 0, -1)
ref_plane "to_Bolt_1_200_ZX" through (226.0766, 0, -250) normal (0, 0, -1) x (0, 1, 0)
ref_plane "to_Bolt_1_201_XY" through (228.4689, 0, -250) normal (0, 1, 0) x (1, 0, 0)
ref_plane "to_Bolt_1_201_YZ" through (228.4689, 0, -250) normal (1, 0, 0) x (0, 0, -1)
ref_plane "to_Bolt_1_201_ZX" through (228.4689, 0, -250) normal (0, 0, -1) x (0, 1, 0)
ref_plane "to_Bolt_1_202_XY" through (230.8612, 0, -250) normal (0, 1, 0) x (1, 0, 0)
ref_plane "to_Bolt_1_202_YZ" through (230.8612, 0, -250) normal (1, 0, 0) x (0, 0, -1)
ref_plane "to_Bolt_1_202_ZX" through (230.8612, 0, -250) normal (0, 0, -1) x (0, 1, 0)
ref_plane "to_Bolt_1_203_XY" through (233.2536, 0, -250) normal (0, 1, 0) x (1, 0, 0)
ref_plane "to_Bolt_1_203_YZ" through (233.2536, 0, -250) normal (1, 0, 0) x (0, 0, -1)
ref_plane "to_Bolt_1_203_ZX" through (233.2536, 0, -250) normal (0, 0, -1) x (0, 1, 0)
ref_plane "to_Bolt_1_204_XY" through (235.6459, 0, -250) normal (0, 1, 0) x (1, 0, 0)
ref_plane "to_Bolt_1_204_YZ" through (235.6459, 0, -250) normal (1, 0, 0) x (0, 0, -1)
ref_plane "to_Bolt_1_204_ZX" through (235.6459, 0, -250) normal (0, 0, -1) x (0, 1, 0)
ref_plane "to_Bolt_1_205_XY" through (238.0383, 0, -250) normal (0, 1, 0) x (1, 0, 0)
ref_plane "to_Bolt_1_205_YZ" through (238.0383, 0, -250) normal (1, 0, 0) x (0, 0, -1)
ref_plane "to_Bolt_1_205_ZX" through (238.0383, 0, -250) normal (0, 0, -1) x (0, 1, 0)
ref_plane "to_Bolt_1_206_XY" through (240.4306, 0, -250) normal (0, 1, 0) x (1, 0, 0)
ref_plane "to_Bolt_1_206_YZ" through (240.4306, 0, -250) normal (1, 0, 0) x (0, 0, -1)
ref_plane "to_Bolt_1_206_ZX" through (240.4306, 0, -250) normal (0, 0, -1) x (0, 1, 0)
ref_plane "to_Bolt_1_207_XY" through (242.823, 0, -250) normal (0, 1, 0) x (1, 0, 0)
ref_plane "to_Bolt_1_207_YZ" through (242.823, 0, -250) normal (1, 0, 0) x (0, 0, -1)
ref_plane "to_Bolt_1_207_ZX" through (242.823, 0, -250) normal (0, 0, -1) x (0, 1, 0)
ref_plane "to_Bolt_1_208_XY" through (245.2153, 0, -250) normal (0, 1, 0) x (1, 0, 0)
ref_plane "to_Bolt_1_208_YZ" through (245.2153, 0, -250) normal (1, 0, 0) x (0, 0, -1)
ref_plane "to_Bolt_1_208_ZX" through (245.2153, 0, -250) normal (0, 0, -1) x (0, 1, 0)
ref_plane "to_Bolt_1_209_XY" through (247.6077, 0, -250) normal (0, 1, 0) x (1, 0, 0)
ref_plane "to_Bolt_1_209_YZ" through (247.6077, 0, -250) normal (1, 0, 0) x (0, 0, -1)
ref_plane "to_Bolt_1_209_ZX" through (247.6077, 0, -250) normal (0, 0, -1) x (0, 1, 0)
ref_plane "to_Bolt_1_21_XY" through (-202.1531, 0, -250) normal (0, 1, 0) x (1, 0, 0)
ref_plane "to_Bolt_1_21_YZ" through (-202.1531, 0, -250) normal (1, 0, 0) x (0, 0, -1)
ref_plane "to_Bolt_1_21_ZX" through (-202.1531, 0, -250) normal (0, 0, -1) x (0, 1, 0)
ref_plane "to_Bolt_1_210_XY" through (250, 0, -250) normal (0, 1, 0) x (1, 0, 0)
ref_plane "to_Bolt_1_210_YZ" through (250, 0, -250) normal (1, 0, 0) x (0, 0, -1)
ref_plane "to_Bolt_1_210_ZX" through (250, 0, -250) normal (0, 0, -1) x (0, 1, 0)
ref_plane "to_Bolt_1_211_XY" through (-250, 0, 250) normal (0, 1, 0) x (1, 0, 0)
ref_plane "to_Bolt_1_211_YZ" through (-250, 0, 250) normal (1, 0, 0) x (0, 0, -1)
ref_plane "to_Bolt_1_211_ZX" through (-250, 0, 250) normal (0, 0, -1) x (0, 1, 0)
ref_plane "to_Bolt_1_212_XY" through (-247.6077, 0, 250) normal (0, 1, 0) x (1, 0, 0)
ref_plane "to_Bolt_1_212_YZ" through (-247.6077, 0, 250) normal (1, 0, 0) x (0, 0, -1)
ref_plane "to_Bolt_1_212_ZX" through (-247.6077, 0, 250) normal (0, 0, -1) x (0, 1, 0)
ref_plane "to_Bolt_1_213_XY" through (-245.2153, 0, 250) normal (0, 1, 0) x (1, 0, 0)
ref_plane "to_Bolt_1_213_YZ" through (-245.2153, 0, 250) normal (1, 0, 0) x (0, 0, -1)
ref_plane "to_Bolt_1_213_ZX" through (-245.2153, 0, 250) normal (0, 0, -1) x (0, 1, 0)
ref_plane "to_Bolt_1_214_XY" through (-248.823, 0, 250) normal (0, 1, 0) x (1, 0, 0)
ref_plane "to_Bolt_1_214_YZ" through (-248.823, 0, 250) normal (1, 0, 0) x (0, 0, -1)
ref_plane "to_Bolt_1_214_ZX" through (-248.823, 0, 250) normal (0, 0, -1) x (0, 1, 0)
ref_plane "to_Bolt_1_215_XY" through (-240.4306, 0, 250) normal (0, 1, 0) x (1, 0, 0)
ref_plane "to_Bolt_1_215_YZ" through (-240.4306, 0, 250) normal (1, 0, 0) x (0, 0, -1)
ref_plane "to_Bolt_1_215_ZX" through (-240.4306, 0, 250) normal (0, 0, -1) x (0, 1, 0)
ref_plane "to_Bolt_1_216_XY" through (-238.0383, 0, 250) normal (0, 1, 0) x (1, 0, 0)
ref_plane "to_Bolt_1_216_YZ" through (-238.0383, 0, 250) normal (1, 0, 0) x (0, 0, -1)
ref_plane "to_Bolt_1_216_ZX" through (-238.0383, 0, 250) normal (0, 0, -1) x (0, 1, 0)
ref_plane "to_Bolt_1_217_XY" through (-235.6459, 0, 250) normal (0, 1, 0) x (1, 0, 0)
ref_plane "to_Bolt_1_217_YZ" through (-235.6459, 0, 250) normal (1, 0, 0) x (0, 0, -1)
ref_plane "to_Bolt_1_217_ZX" through (-235.6459, 0, 250) normal (0, 0, -1) x (0, 1, 0)
ref_plane "to_Bolt_1_218_XY" through (-233.2536, 0, 250) normal (0, 1, 0) x (1, 0, 0)
ref_plane "to_Bolt_1_218_YZ" through (-233.2536, 0, 250) normal (1, 0, 0) x (0, 0, -1)
ref_plane "to_Bolt_1_218_ZX" through (-233.2536, 0, 250) normal (0, 0, -1) x (0, 1, 0)
ref_plane "to_Bolt_1_219_XY" through (-230.8612, 0, 250) normal (0, 1, 0) x (1, 0, 0)
ref_plane "to_Bolt_1_219_YZ" through (-230.8612, 0, 250) normal (1, 0, 0) x (0, 0, -1)
ref_plane "to_Bolt_1_219_ZX" through (-230.8612, 0, 250) normal (0, 0, -1) x (0, 1, 0)
ref_plane "to_Bolt_1_22_XY" through (-199.7608, 0, -250) normal (0, 1, 0) x (1, 0, 0)
ref_plane "to_Bolt_1_22_YZ" through (-199.7608, 0, -250) normal (1, 0, 0) x (0, 0, -1)
ref_plane "to_Bolt_1_22_ZX" through (-199.7608, 0, -250) normal (0, 0, -1) x (0, 1, 0)
ref_plane "to_Bolt_1_220_XY" through (-228.4689, 0, 250) normal (0, 1, 0) x (1, 0, 0)
ref_plane "to_Bolt_1_220_YZ" through (-228.4689, 0, 250) normal (1, 0, 0) x (0, 0, -1)
ref_plane "to_Bolt_1_220_ZX" through (-228.4689, 0, 250) normal (0, 0, -1) x (0, 1, 0)
ref_plane "to_Bolt_1_221_XY" through (-226.0766, 0, 250) normal (0, 1, 0) x (1, 0, 0)
ref_plane "to_Bolt_1_221_YZ" through (-226.0766, 0, 250) normal (1, 0, 0) x (0, 0, -1)
ref_plane "to_Bolt_1_221_ZX" through (-226.0766, 0, 250) normal (0, 0, -1) x (0, 1, 0)
ref_plane "to_Bolt_1_222_XY" through (-223.6842, 0, 250) normal (0, 1, 0) x (1, 0, 0)
ref_plane "to_Bolt_1_222_YZ" through (-223.6842, 0, 250) normal (1, 0, 0) x (0, 0, -1)
ref_plane "to_Bolt_1_222_ZX" through (-223.6842, 0, 250) normal (0, 0, -1) x (0, 1, 0)
ref_plane "to_Bolt_1_223_XY" through (-221.2919, 0, 250) normal (0, 1, 0) x (1, 0, 0)
ref_plane "to_Bolt_1_223_YZ" through (-221.2919, 0, 250) normal (1, 0, 0) x (0, 0, -1)
ref_plane "to_Bolt_1_223_ZX" through (-221.2919, 0, 250) normal (0, 0, -1) x (0, 1, 0)
ref_plane "to_Bolt_1_224_XY" through (-218.8995, 0, 250) normal (0, 1, 0) x (1, 0, 0)
ref_plane "to_Bolt_1_224_YZ" through (-218.8995, 0, 250) normal (1, 0, 0) x (0, 0, -1)
ref_plane "to_Bolt_1_224_ZX" through (-218.8995, 0, 250) normal (0, 0, -1) x (0, 1, 0)
ref_plane "to_Bolt_1_225_XY" through (-216.5072, 0, 250) normal (0, 1, 0) x (1, 0, 0)
ref_plane "to_Bolt_1_225_YZ" through (-216.5072, 0, 250) normal (1, 0, 0) x (0, 0, -1)
ref_plane "to_Bolt_1_225_ZX" through (-216.5072, 0, 250) normal (0, 0, -1) x (0, 1, 0)
ref_plane "to_Bolt_1_226_XY" through (-214.1148, 0, 250) normal (0, 1, 0) x (1, 0, 0)
ref_plane "to_Bolt_1_226_YZ" through (-214.1148, 0, 250) normal (1, 0, 0) x (0, 0, -1)
ref_plane "to_Bolt_1_226_ZX" through (-214.1148, 0, 250) normal (0, 0, -1) x (0, 1, 0)
ref_plane "to_Bolt_1_227_XY" through (-211.7225, 0, 250) normal (0, 1, 0) x (1, 0, 0)
ref_plane "to_Bolt_1_227_YZ" through (-211.7225, 0, 250) normal (1, 0, 0) x (0, 0, -1)
ref_plane "to_Bolt_1_227_ZX" through (-211.7225, 0, 250) normal (0, 0, -1) x (0, 1, 0)
ref_plane "to_Bolt_1_228_XY" through (-209.3301, 0, 250) normal (0, 1, 0) x (1, 0, 0)
ref_plane "to_Bolt_1_228_YZ" through (-209.3301, 0, 250) normal (1, 0, 0) x (0, 0, -1)
ref_plane "to_Bolt_1_228_ZX" through (-209.3301, 0, 250) normal (0, 0, -1) x (0, 1, 0)
ref_plane "to_Bolt_1_229_XY" through (-206.9378, 0, 250) normal (0, 1, 0) x (1, 0, 0)
ref_plane "to_Bolt_1_229_YZ" through (-206.9378, 0, 250) normal (1, 0, 0) x (0, 0, -1)
ref_plane "to_Bolt_1_229_ZX" through (-206.9378, 0, 250) normal (0, 0, -1) x (0, 1, 0)
ref_plane "to_Bolt_1_23_XY" through (-197.3684, 0, -250) normal (0, 1, 0) x (1, 0, 0)
ref_plane "to_Bolt_1_23_YZ" through (-197.3684, 0, -250) normal (1, 0, 0) x (0, 0, -1)
ref_plane "to_Bolt_1_23_ZX" through (-197.3684, 0, -250) normal (0, 0, -1) x (0, 1, 0)
ref_plane "to_Bolt_1_230_XY" through (-204.5455, 0, 250) normal (0, 1, 0) x (1, 0, 0)
ref_plane "to_Bolt_1_230_YZ" through (-204.5455, 0, 250) normal (1, 0, 0) x (0, 0, -1)
ref_plane "to_Bolt_1_230_ZX" through (-204.5455, 0, 250) normal (0, 0, -1) x (0, 1, 0)
ref_plane "to_Bolt_1_231_XY" through (-202.1531, 0, 250) normal (0, 1, 0) x (1, 0, 0)
ref_plane "to_Bolt_1_231_YZ" through (-202.1531, 0, 250) normal (1, 0, 0) x (0, 0, -1)
ref_plane "to_Bolt_1_231_ZX" through (-202.1531, 0, 250) normal (0, 0, -1) x (0, 1, 0)
ref_plane "to_Bolt_1_232_XY" through (-199.7608, 0, 250) normal (0, 1, 0) x (1, 0, 0)
ref_plane "to_Bolt_1_232_YZ" through (-199.7608, 0, 250) normal (1, 0, 0) x (0, 0, -1)
ref_plane "to_Bolt_1_232_ZX" through (-199.7608, 0, 250) normal (0, 0, -1) x (0, 1, 0)
ref_plane "to_Bolt_1_233_XY" through (-197.3684, 0, 250) normal (0, 1, 0) x (1, 0, 0)
ref_plane "to_Bolt_1_233_YZ" through (-197.3684, 0, 250) normal (1, 0, 0) x (0, 0, -1)
ref_plane "to_Bolt_1_233_ZX" through (-197.3684, 0, 250) normal (0, 0, -1) x (0, 1, 0)
ref_plane "to_Bolt_1_234_XY" through (-194.9761, 0, 250) normal (0, 1, 0) x (1, 0, 0)
ref_plane "to_Bolt_1_234_YZ" through (-194.9761, 0, 250) normal (1, 0, 0) x (0, 0, -1)
ref_plane "to_Bolt_1_234_ZX" through (-194.9761, 0, 250) normal (0, 0, -1) x (0, 1, 0)
ref_plane "to_Bolt_1_235_XY" through (-192.5837, 0, 250) normal (0, 1, 0) x (1, 0, 0)
ref_plane "to_Bolt_1_235_YZ" through (-192.5837, 0, 250) normal (1, 0, 0) x (0, 0, -1)
ref_plane "to_Bolt_1_235_ZX" through (-192.5837, 0, 250) normal (0, 0, -1) x (0, 1, 0)
ref_plane "to_Bolt_1_236_XY" through (-190.1914, 0, 250) normal (0, 1, 0) x (1, 0, 0)
ref_plane "to_Bolt_1_236_YZ" through (-190.1914, 0, 250) normal (1, 0, 0) x (0, 0, -1)
ref_plane "to_Bolt_1_236_ZX" through (-190.1914, 0, 250) normal (0, 0, -1) x (0, 1, 0)
ref_plane "to_Bolt_1_237_XY" through (-187.799, 0, 250) normal (0, 1, 0) x (1, 0, 0)
ref_plane "to_Bolt_1_237_YZ" through (-187.799, 0, 250) normal (1, 0, 0) x (0, 0, -1)
ref_plane "to_Bolt_1_237_ZX" through (-187.799, 0, 250) normal (0, 0, -1) x (0, 1, 0)
ref_plane "to_Bolt_1_238_XY" through (-185.4067, 0, 250) normal (0, 1, 0) x (1, 0, 0)
ref_plane "to_Bolt_1_238_YZ" through (-185.4067, 0, 250) normal (1, 0, 0) x (0, 0, -1)
ref_plane "to_Bolt_1_238_ZX" through (-185.4067, 0, 250) normal (0, 0, -1) x (0, 1, 0)
ref_plane "to_Bolt_1_239_XY" through (-183.0144, 0, 250) normal (0, 1, 0) x (1, 0, 0)
ref_plane "to_Bolt_1_239_YZ" through (-183.0144, 0, 250) normal (1, 0, 0) x (0, 0, -1)
ref_plane "to_Bolt_1_239_ZX" through (-183.0144, 0, 250) normal (0, 0, -1) x (0, 1, 0)
ref_plane "to_Bolt_1_24_XY" through (-194.9761, 0, -250) normal (0, 1, 0) x (1, 0, 0)
ref_plane "to_Bolt_1_24_YZ" through (-194.9761, 0, -250) normal (1, 0, 0) x (0, 0, -1)
ref_plane "to_Bolt_1_24_ZX" through (-194.9761, 0, -250) normal (0, 0, -1) x (0, 1, 0)
ref_plane "to_Bolt_1_240_XY" through (-180.622, 0, 250) normal (0, 1, 0) x (1, 0, 0)
ref_plane "to_Bolt_1_240_YZ" through (-180.622, 0, 250) normal (1, 0, 0) x (0, 0, -1)
ref_plane "to_Bolt_1_240_ZX" through (-180.622, 0, 250) normal (0, 0, -1) x (0, 1, 0)
ref_plane "to_Bolt_1_241_XY" through (-178.2297, 0, 250) normal (0, 1, 0) x (1, 0, 0)
ref_plane "to_Bolt_1_241_YZ" through (-178.2297, 0, 250) normal (1, 0, 0) x (0, 0, -1)
ref_plane "to_Bolt_1_241_ZX" through (-178.2297, 0, 250) normal (0, 0, -1) x (0, 1, 0)
ref_plane "to_Bolt_1_242_XY" through (-175.8373, 0, 250) normal (0, 1, 0) x (1, 0, 0)
ref_plane "to_Bolt_1_242_YZ" through (-175.8373, 0, 250) normal (1, 0, 0) x (0, 0, -1)
ref_plane "to_Bolt_1_242_ZX" through (-175.8373, 0, 250) normal (0, 0, -1) x (0, 1, 0)
ref_plane "to_Bolt_1_243_XY" through (-173.445, 0, 250) normal (0, 1, 0) x (1, 0, 0)
ref_plane "to_Bolt_1_243_YZ" through (-173.445, 0, 250) normal (1, 0, 0) x (0, 0, -1)
ref_plane "to_Bolt_1_243_ZX" through (-173.445, 0, 250) normal (0, 0, -1) x (0, 1, 0)
ref_plane "to_Bolt_1_244_XY" through (-171.0526, 0, 250) normal (0, 1, 0) x (1, 0, 0)
ref_plane "to_Bolt_1_244_YZ" through (-171.0526, 0, 250) normal (1, 0, 0) x (0, 0, -1)
ref_plane "to_Bolt_1_244_ZX" through (-171.0526, 0, 250) normal (0, 0, -1) x (0, 1, 0)
ref_plane "to_Bolt_1_245_XY" through (-168.6603, 0, 250) normal (0, 1, 0) x (1, 0, 0)
ref_plane "to_Bolt_1_245_YZ" through (-168.6603, 0, 250) normal (1, 0, 0) x (0, 0, -1)
ref_plane "to_Bolt_1_245_ZX" through (-168.6603, 0, 250) normal (0, 0, -1) x (0, 1, 0)
ref_plane "to_Bolt_1_246_XY" through (-166.2679, 0, 250) normal (0, 1, 0) x (1, 0, 0)
ref_plane "to_Bolt_1_246_YZ" through (-166.2679, 0, 250) normal (1, 0, 0) x (0, 0, -1)
ref_plane "to_Bolt_1_246_ZX" through (-166.2679, 0, 250) normal (0, 0, -1) x (0, 1, 0)
ref_plane "to_Bolt_1_247_XY" through (-163.8756, 0, 250) normal (0, 1, 0) x (1, 0, 0)
ref_plane "to_Bolt_1_247_YZ" through (-163.8756, 0, 250) normal (1, 0, 0) x (0, 0, -1)
ref_plane "to_Bolt_1_247_ZX" through (-163.8756, 0, 250) normal (0, 0, -1) x (0, 1, 0)
ref_plane "to_Bolt_1_248_XY" through (-161.4833, 0, 250) normal (0, 1, 0) x (1, 0, 0)
ref_plane "to_Bolt_1_248_YZ" through (-161.4833, 0, 250) normal (1, 0, 0) x (0, 0, -1)
ref_plane "to_Bolt_1_248_ZX" through (-161.4833, 0, 250) normal (0, 0, -1) x (0, 1, 0)
ref_plane "to_Bolt_1_249_XY" through (-159.0909, 0, 250) normal (0, 1, 0) x (1, 0, 0)
ref_plane "to_Bolt_1_249_YZ" through (-159.0909, 0, 250) normal (1, 0, 0) x (0, 0, -1)
ref_plane "to_Bolt_1_249_ZX" through (-159.0909, 0, 250) normal (0, 0, -1) x (0, 1, 0)
ref_plane "to_Bolt_1_25_XY" through (-192.5837, 0, -250) normal (0, 1, 0) x (1, 0, 0)
ref_plane "to_Bolt_1_25_YZ" through (-192.5837, 0, -250) normal (1, 0, 0) x (0, 0, -1)
ref_plane "to_Bolt_1_25_ZX" through (-192.5837, 0, -250) normal (0, 0, -1) x (0, 1, 0)
ref_plane "to_Bolt_1_250_XY" through (-156.6986, 0, 250) normal (0, 1, 0) x (1, 0, 0)
ref_plane "to_Bolt_1_250_YZ" through (-156.6986, 0, 250) normal (1, 0, 0) x (0, 0, -1)
ref_plane "to_Bolt_1_250_ZX" through (-156.6986, 0, 250) normal (0, 0, -1) x (0, 1, 0)
ref_plane "to_Bolt_1_251_XY" through (-154.3062, 0, 250) normal (0, 1, 0) x (1, 0, 0)
ref_plane "to_Bolt_1_251_YZ" through (-154.3062, 0, 250) normal (1, 0, 0) x (0, 0, -1)
ref_plane "to_Bolt_1_251_ZX" through (-154.3062, 0, 250) normal (0, 0, -1) x (0, 1, 0)
ref_plane "to_Bolt_1_252_XY" through (-151.9139, 0, 250) normal (0, 1, 0) x (1, 0, 0)
ref_plane "to_Bolt_1_252_YZ" through (-151.9139, 0, 250) normal (1, 0, 0) x (0, 0, -1)
ref_plane "to_Bolt_1_252_ZX" through (-151.9139, 0, 250) normal (0, 0, -1) x (0, 1, 0)
ref_plane "to_Bolt_1_253_XY" through (-149.5215, 0, 250) normal (0, 1, 0) x (1, 0, 0)
ref_plane "to_Bolt_1_253_YZ" through (-149.5215, 0, 250) normal (1, 0, 0) x (0, 0, -1)
ref_plane "to_Bolt_1_253_ZX" through (-149.5215, 0, 250) normal (0, 0, -1) x (0, 1, 0)
ref_plane "to_Bolt_1_254_XY" through (-147.1292, 0, 250) normal (0, 1, 0) x (1, 0, 0)
ref_plane "to_Bolt_1_254_YZ" through (-147.1292, 0, 250) normal (1, 0, 0) x (0, 0, -1)
ref_plane "to_Bolt_1_254_ZX" through (-147.1292, 0, 250) normal (0, 0, -1) x (0, 1, 0)
ref_plane "to_Bolt_1_255_XY" through (-144.7368, 0, 250) normal (0, 1, 0) x (1, 0, 0)
ref_plane "to_Bolt_1_255_YZ" through (-144.7368, 0, 250) normal (1, 0, 0) x (0, 0, -1)
ref_plane "to_Bolt_1_255_ZX" through (-144.7368, 0, 250) normal (0, 0, -1) x (0, 1, 0)
ref_plane "to_Bolt_1_256_XY" through (-142.3445, 0, 250) normal (0, 1, 0) x (1, 0, 0)
ref_plane "to_Bolt_1_256_YZ" through (-142.3445, 0, 250) normal (1, 0, 0) x (0, 0, -1)
ref_plane "to_Bolt_1_256_ZX" through (-142.3445, 0, 250) normal (0, 0, -1) x (0, 1, 0)
ref_plane "to_Bolt_1_257_XY" through (-139.9522, 0, 250) normal (0, 1, 0) x (1, 0, 0)
ref_plane "to_Bolt_1_257_YZ" through (-139.9522, 0, 250) normal (1, 0, 0) x (0, 0, -1)
ref_plane "to_Bolt_1_257_ZX" through (-139.9522, 0, 250) normal (0, 0, -1) x (0, 1, 0)
ref_plane "to_Bolt_1_258_XY" through (-137.5598, 0, 250) normal (0, 1, 0) x (1, 0, 0)
ref_plane "to_Bolt_1_258_YZ" through (-137.5598, 0, 250) normal (1, 0, 0) x (0, 0, -1)
ref_plane "to_Bolt_1_258_ZX" through (-137.5598, 0, 250) normal (0, 0, -1) x (0, 1, 0)
ref_plane "to_Bolt_1_259_XY" through (-135.1675, 0, 250) normal (0, 1, 0) x (1, 0, 0)
ref_plane "to_Bolt_1_259_YZ" through (-135.1675, 0, 250) normal (1, 0, 0) x (0, 0, -1)
ref_plane "to_Bolt_1_259_ZX" through (-135.1675, 0, 250) normal (0, 0, -1) x (0, 1, 0)
ref_plane "to_Bolt_1_26_XY" through (-190.1914, 0, -250) normal (0, 1, 0) x (1, 0, 0)
ref_plane "to_Bolt_1_26_YZ" through (-190.1914, 0, -250) normal (1, 0, 0) x (0, 0, -1)